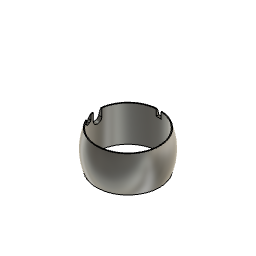
sphere_PS4 v1 (Autodesk Fusion 360 design; units mm, degrees)
Autodesk Fusion 360 part; units mm, degrees
note: some values were not read from the file. Set by a fixed rule: which sketch regions a step uses.
ref_plane "Arbeitsebene2" through (0, 0, 70) normal (0, 0, 1) x (1, 0, 0)
sketch "Skizze1" plane through (0, 0, 70) normal (0, 0, 1) x (1, 0, 0)
  circle A0 centre (0, 0) radius 60
  line L0 (-32, -65.4497) -> (-32, 74.1763) construction
  line L1 (32, -65.9786) -> (32, 70) construction
  line L2 (-70, -45) -> (87.8831, -45) construction
  line L3 (-67.6095, 45) -> (98.1964, 45) construction
  line L4 (-42.2555, 59.4219) -> (47.2161, -66.3977) construction
  line L5 (-55.8567, -78.5485) -> (54.1174, 76.1026) construction
  line L6 (4.6, 47.5) -> (-4.6, 47.5)
  line L7 (-4.6, 47.5) -> (-4.6, 72.5)
  line L8 (-4.6, 72.5) -> (4.6, 72.5)
  line L9 (4.6, 72.5) -> (4.6, 47.5)
  line L10 (4.6, 47.5) -> (-4.6, 72.5) construction
  line L11 (-4.6, 47.5) -> (4.6, 72.5) construction
  line L12 (0, 80.8433) -> (0, -85.8515) construction
  line L13 (-51.741, 47.0895) -> (-51.741, -61.7465) construction
  line L14 (18.5366, 6.8393) -> (-95.6456, -35.2896) construction
  line L15 (-71.1394, 33.485) -> (-36.9267, -59.2417) construction
  point P0 (-32, 45)
  point P1 (32, -45)
  point P2 (-32, -45)
  point P3 (34.8015, 48.8759)
  point P4 (32, 45)
  point P5 (0, 60)
  point P6 (-51.741, -19.0905)
  dimension "d1" = 120
  dimension "d8" = 45
  dimension "d9" = 45
  dimension "d10" = 32
  dimension "d11" = 32
  dimension "d24" = 9.2
  dimension "d25" = 25
  dimension "d38" = 51.741
  dimension "d39" = 19.0905
  constraint coincident A0.centre origin
  constraint vertical L0
  constraint vertical L1
  constraint horizontal L2
  constraint perpendicular L1 L3
  constraint coincident A0.centre L4
  constraint coincident L0 P0
  constraint coincident L3 P0
  constraint coincident L2 P1
  constraint coincident L1 P1
  constraint coincident L0 P2
  constraint coincident L2 P2
  constraint coincident L4 P0
  constraint coincident A0.centre L5
  constraint coincident A0 P3
  constraint coincident L1 P4
  constraint coincident L3 P4
  constraint coincident L5 P4
  constraint horizontal L6
  constraint perpendicular L6 L7
  constraint parallel L6 L8
  constraint parallel L7 L9
  constraint coincident L10 P5
  constraint coincident L11 P5
  constraint vertical L12
  constraint coincident A0.centre L12
  constraint coincident P5 L12
  constraint coincident A0 P5
  constraint vertical L13
  constraint coincident L13 P6
  constraint coincident P6 L14
  constraint coincident A0.centre L14
  constraint perpendicular L14 L15
  constraint coincident P6 L15
  measures "d1" diameter of A0
  measures "d8" distance of A0.centre L3
  measures "d9" distance of A0.centre L2
  measures "d10" distance of A0.centre L1
  measures "d11" distance of A0.centre L0
  measures "d24" distance of L7 L9
  measures "d25" distance of L6 L8
  measures "d38" distance of A0.centre L13
  measures "d39" vertical distance of A0.centre P6
sketch "Skizze4" plane through (0, 0, 0) normal (0, 1, 0) x (1, 0, 0)
  line L0 (-48.1569, -35) -> (99.3062, -35) construction
  line L1 (60.1, -70) -> (60.1, 0)
  line L2 (60.1, 0) -> (61.6, 0)
  arc A0 (61.6, -70) -> (61.6, 0) centre (-32.075, -35) ccw
  line L3 (60.1, -70) -> (61.6, -70)
  point P0 (-32.075, -35)
  dimension "d31" = 35
  dimension "d32" = 60.1
  dimension "d33" = 1.5
  dimension "d34" = 35
  dimension "d35" = 1.5
  dimension "d36" = 100
  constraint horizontal L0
  constraint perpendicular L0 L1
  constraint horizontal L2
  constraint coincident origin L2
  constraint coincident L1.end L2.start
  constraint coincident L0 P0
  constraint coincident P0 A0.centre
  constraint horizontal L3
  constraint coincident L1.start L3.start
  constraint coincident A0.start L3.end
  measures "d31" distance of origin L0
  measures "d32" distance of origin L1
  measures "d33" distance of L1.end L2.end
  measures "d34" distance of L0 L3
  measures "d35" distance of L1.start A0.start
  measures "d36" radius of A0
revolve "Drehen2" add sketch "Skizze4" angle 360 about axis through (0, 0, 1.75) along (0, 0, 1)
ref_plane "Arbeitsebene3" through (-51.741, -19.0905, 70) normal (0.938178, 0.346153, 0) x (-0.346153, 0.938178, 0)
sketch "Skizze5" plane through (-51.741, -19.0905, 0) normal (0.938178, 0.346153, 0) x (-0.346153, 0.938178, 0)
  line L0 (22.1819, 62) -> (-34.0583, 62) construction
  line L1 (45.7665, 70) -> (-50, 70) construction
  line L2 (60, 70) -> (-60, 70)
  line L3 (0, -62.5) -> (0, 202.5)
  line L4 (-4, 59) -> (4, 59)
  line L5 (7, 70) -> (-29, 70)
  line L6 (-7, 70) -> (-7, 62)
  line L7 (7, 70) -> (7, 62)
  arc A0 (4, 59) -> (7, 62) centre (4, 62) ccw
  arc A1 (-7, 62) -> (-4, 59) centre (-4, 62) ccw
  point P0 (4, 62)
  point P1 (-4, 62)
  point P2 (0, 70)
  point P3 (0, 70)
  dimension "d40" = 70
  dimension "d41" = 8
  dimension "d44" = 4
  dimension "d45" = 4
  constraint horizontal L0
  constraint horizontal L1
  constraint horizontal L4
  constraint horizontal L5
  constraint coincident L1 P3
  constraint coincident L3 P3
  constraint coincident L5 P3
  constraint vertical L6
  constraint vertical L7
  constraint coincident L0 P1
  constraint coincident L2 L6.start
  constraint coincident L2 L5.start
  constraint coincident L5.start L7.start
  constraint coincident P0 A0.centre
  constraint coincident P1 A1.centre
  measures "d40" distance of origin L1
  measures "d41" distance of L0 L2
  measures "d44" distance of L3 P0
  measures "d45" distance of L3 P1
extrude "Extrusion1" cut sketch "Skizze5" along normal mid plane 40
extrude "Extrusion2" cut sketch "Skizze1" against normal blind 12.5 contours A0 L6 L7 L9 | A0 L7 L8 L9 picked at (-1.4809, 11.7216)
sketch "Skizze6" plane through (0, 0, 0) normal (1, 0, 0) x (0, 1, 0)
  line L0 (8.2, 70) -> (-95.5036, 70) construction
  line L1 (8.2, 70) -> (8.2, 55)
  line L2 (-8.2, 70) -> (-8.2, 55)
  line L3 (0, 78.2576) -> (0, 37.1704) construction
  line L4 (52.1379, 70) -> (-8.2, 70)
  arc A0 (-8.2, 55) -> (8.2, 55) centre (0, 55) ccw
  point P0 (0, 55)
  dimension "d50" = 70
  dimension "d51" = 8.2
  dimension "d52" = 8.2
  dimension "d54" = 15
  constraint horizontal L0
  constraint perpendicular L0 L1
  constraint perpendicular L0 L2
  constraint perpendicular L0 L3
  constraint coincident origin L3
  constraint coincident L0 L1.start
  constraint coincident L0 L2.start
  constraint horizontal L4
  constraint coincident L2.start L4.end
  constraint coincident L0.start L1.start
  constraint coincident P0 A0.centre
  measures "d50" distance of origin L0
  measures "d51" distance of origin L2
  measures "d52" distance of origin L1
  measures "d54" distance of L0 P0
extrude "Extrusion3" cut sketch "Skizze6" against normal blind 90
